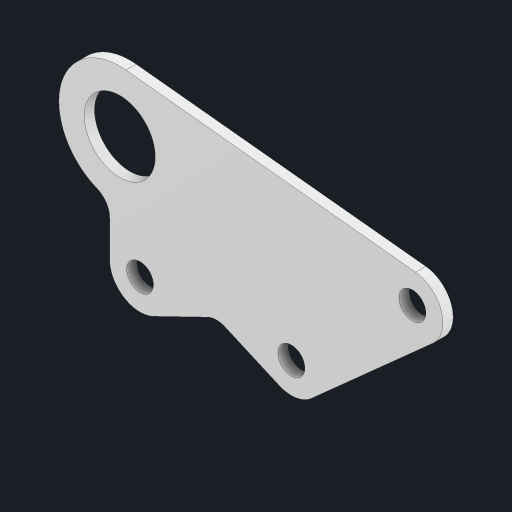
# Autodesk Inventor part: gear_gusset
Saved by Autodesk Inventor 2024 (Build 280153000, 153)
## iProperties
Created: 2023-08-16
Part Number: gear_gusset
Material: Acetal Resin, White
Document SubType Name: Modeling
Designer: avere
Density: 1.425 g/cm^3
Appearance: Smooth - White
Author: avere
Autodesk Inventor part; units mm, degrees
ref_plane "YZ Plane" through (0, 0, 0) normal (1, 0, 0) x (0, 1, 0)
ref_plane "XZ Plane" through (0, 0, 0) normal (0, 1, 0) x (-1, 0, 0)
ref_plane "XY Plane" through (0, 0, 0) normal (0, 0, 1) x (1, 0, 0)
sketch "Sketch1" plane through (0, 0, 0) normal (0, 0, 1) x (1, 0, 0)
  circle A0 centre (0, 0) radius 5.5499
  circle A1 centre (45.7905, 0) radius 2.0955
  circle A2 centre (26.8579, -16.9327) radius 2.0955
  arc A3 (0.9907, 9.4733) -> (-3.8129, -8.7285) centre (0, 0) ccw
  arc A4 (48.9628, -3.5521) -> (46.2858, 4.7367) centre (45.7905, 0) ccw
  arc A5 (24.9354, -21.2869) -> (30.0142, -20.4747) centre (26.8419, -16.9226) ccw
  line L0 (0.9907, 9.4733) -> (46.2858, 4.7367)
  line L1 (30.0142, -20.4747) -> (48.9628, -3.5521)
  line L2 (-3.8129, -8.7285) -> (24.9354, -21.2869)
  dimension "d0" = 11.0998
  dimension "d12" = 4.191
  dimension "d15" = 4.191
  dimension "d16" = 19.05
  dimension "d17" = 9.525
  dimension "d18" = 9.525
  constraints: 6 centre point, 6 end point, 6 point on circle, 6 tangent, 2 coincident
  measures "d0" diameter of A0
  measures "d12" diameter of A1
  measures "d15" diameter of A2
  measures "d16" diameter of A3
  measures "d17" diameter of A4
  measures "d18" diameter of A5
extrude "Extrusion1" add sketch "Sketch1" along normal blind 1.5875
sketch "Sketch2" plane through (0, 0, 1.5875) normal (0, 0, 1) x (1, 0, 0)
  circle A0 centre (3.175, -17.4625) radius 2.0828
  arc A1 (-1.5875, -17.4625) -> (5.2577, -21.7454) centre (3.175, -17.4625) ccw
  line L0 (-1.5875, -17.4625) -> (-1.5875, -11.7784)
  line L1 (-3.8129, -8.7285) -> (24.9354, -21.2869) projected
  arc A2 (-1.5875, -11.7784) -> (-3.4915, -8.8689) centre (-4.7625, -11.7784) ccw
  line L2 (5.2577, -21.7454) -> (13.7491, -17.6162)
  arc A3 (24.9354, -21.2869) -> (30.0142, -20.4747) centre (26.8419, -16.9226) ccw projected
  arc A4 (16.4085, -17.562) -> (13.7491, -17.6162) centre (15.1376, -20.4715) ccw
  point P0 (0, 0)
  point P1 (-1.5875, -9.7007)
  point P2 (15.0663, -16.9757)
  dimension "d19" = 4.1656
  dimension "d20" = 3.175
  dimension "d21" = 3.175
  constraints: 6 point on circle, 4 centre point, 4 end point, 4 point on line, 4 tangent, 1 coincident, 1 other
  measures "d19" diameter of A0
  measures "d20" radius of A2
  measures "d21" radius of A4
extrude "Extrusion2" add sketch "Sketch2" against normal blind 1.5875
body "Solid1"
